Autodesk Inventor part; units mm, degrees
(part 2 of 2)
sketch "スケッチ2" plane through (0, 0, 2.8) normal (0, 0, 1) x (1, 0, 0)
  arc A0 (151.9662, 105.75) -> (150.8837, 107.625) centre (150.8837, 106.375) ccw
  arc A1 (151.9662, 105.75) -> (151.9662, 104.25) centre (153.2652, 105) ccw
  arc A2 (150.8837, 102.375) -> (151.9662, 104.25) centre (150.8837, 103.625) ccw
  arc A3 (147.4196, 101.625) -> (149.5846, 101.625) centre (148.5021, 102.25) ccw
  arc A4 (150.8837, 102.375) -> (149.5846, 101.625) centre (150.8837, 100.875) ccw
  arc A5 (147.4196, 101.625) -> (146.1205, 102.375) centre (146.1205, 100.875) ccw
  arc A6 (146.1205, 107.625) -> (145.038, 105.75) centre (146.1205, 106.375) ccw
  arc A7 (146.1205, 107.625) -> (147.4196, 108.375) centre (146.1205, 109.125) ccw
  line L0 (145.038, 107) -> (148.5021, 109) construction
  circle A8 centre (148.5021, 105) radius 5
  arc A9 (149.5846, 108.375) -> (147.4196, 108.375) centre (148.5021, 107.75) ccw
  arc A10 (145.038, 104.25) -> (145.038, 105.75) centre (143.739, 105) ccw
  arc A11 (149.5846, 108.375) -> (150.8837, 107.625) centre (150.8837, 109.125) ccw
  line L1 (145.038, 103) -> (145.038, 107) construction
  arc A12 (145.038, 104.25) -> (146.1205, 102.375) centre (146.1205, 103.625) ccw
  line L2 (148.5021, 109) -> (151.9662, 107) construction
  line L3 (148.5021, 101) -> (145.038, 103) construction
  circle A13 centre (148.5021, 105) radius 4 construction
  circle A14 centre (148.5021, 105) radius 3.2631 construction
  line L4 (151.9662, 103) -> (148.5021, 101) construction
  line L5 (151.9662, 107) -> (151.9662, 103) construction
  arc A15 (148.8935, 75.5025) -> (149.2852, 76.5042) centre (138.7786, 80.035) ccw projected
  arc A16 (149.2852, 76.5042) -> (149.4997, 77.2537) centre (141.1512, 79.2377) ccw projected
  arc A17 (149.4997, 77.2537) -> (149.5998, 77.772) centre (143.4588, 78.6893) ccw projected
  arc A18 (149.5998, 77.772) -> (150.4063, 77.8165) centre (148.5021, 105) ccw projected
  arc A19 (150.4063, 77.8165) -> (150.5629, 77.3123) centre (156.4092, 79.4038) ccw projected
  arc A20 (150.5629, 77.3123) -> (150.8585, 76.591) centre (158.6424, 80.2027) ccw projected
  arc A21 (150.8585, 76.591) -> (151.358, 75.6385) centre (160.9129, 81.2562) ccw projected
  arc A22 (151.358, 75.6385) -> (152.1361, 75.7246) centre (148.5021, 105) ccw projected
  arc A23 (152.1361, 75.7246) -> (152.4152, 76.7633) centre (141.584, 79.1169) ccw projected
  arc A24 (152.4152, 76.7633) -> (152.546, 77.5318) centre (144.0299, 78.5854) ccw projected
  arc A25 (152.546, 77.5318) -> (152.5884, 78.0581) centre (146.3838, 78.2942) ccw projected
  arc A26 (152.5884, 78.0581) -> (153.3852, 78.191) centre (148.5021, 105) ccw projected
  arc A27 (153.3852, 78.191) -> (153.5962, 77.7071) centre (159.177, 80.429) ccw projected
  arc A28 (153.5962, 77.7071) -> (153.9695, 77.0227) centre (161.3088, 81.4687) ccw projected
  arc A29 (153.9695, 77.0227) -> (154.5707, 76.1309) centre (163.4496, 82.7656) ccw projected
  arc A30 (154.5707, 76.1309) -> (155.3346, 76.3021) centre (148.5021, 105) ccw projected
  arc A31 (155.3346, 76.3021) -> (155.4977, 77.3651) centre (144.4733, 78.5129) ccw projected
  arc A32 (155.4977, 77.3651) -> (155.5431, 78.1434) centre (146.9629, 78.2537) ccw projected
  arc A33 (155.5431, 78.1434) -> (155.5275, 78.6711) centre (149.3345, 78.2232) ccw projected
  arc A34 (155.5275, 78.6711) -> (156.3048, 78.8909) centre (148.5021, 105) ccw projected
  arc A35 (156.3048, 78.8909) -> (156.5678, 78.4331) centre (161.8152, 81.7524) ccw projected
  arc A36 (156.5678, 78.4331) -> (157.014, 77.7939) centre (163.8197, 83.0204) ccw projected
  arc A37 (157.014, 77.7939) -> (157.7097, 76.9737) centre (165.8049, 84.5449) ccw projected
  arc A38 (157.7097, 76.9737) -> (158.4501, 77.2279) centre (148.5021, 105) ccw projected
  arc A39 (158.4501, 77.2279) -> (158.4953, 78.3024) centre (147.4116, 78.2305) ccw projected
  arc A40 (158.4953, 78.3024) -> (158.4549, 79.081) centre (149.9145, 78.2467) ccw projected
  arc A41 (158.4549, 79.081) -> (158.3812, 79.6038) centre (152.2752, 78.4773) ccw projected
  arc A42 (158.3812, 79.6038) -> (159.1296, 79.9077) centre (148.5021, 105) ccw projected
  arc A43 (159.1296, 79.9077) -> (159.4414, 79.4817) centre (164.2918, 83.3581) ccw projected
  arc A44 (159.4414, 79.4817) -> (159.9553, 78.8954) centre (166.1447, 84.8389) ccw projected
  arc A45 (159.9553, 78.8954) -> (160.737, 78.1567) centre (167.9501, 86.5725) ccw projected
  arc A46 (160.737, 78.1567) -> (161.4449, 78.4908) centre (148.5021, 105) ccw projected
  arc A47 (161.4449, 78.4908) -> (161.3716, 79.5638) centre (150.3631, 78.273) ccw projected
  arc A48 (161.3716, 79.5638) -> (161.2458, 80.3332) centre (152.849, 78.5645) ccw projected
  arc A49 (161.2458, 80.3332) -> (161.1151, 80.8447) centre (155.17, 79.0534) ccw projected
  arc A50 (161.1151, 80.8447) -> (161.8255, 81.2291) centre (148.5021, 105) ccw projected
  arc A51 (161.8255, 81.2291) -> (162.1822, 80.84) centre (166.5768, 85.2264) ccw projected
  arc A52 (162.1822, 80.84) -> (162.7575, 80.3138) centre (168.2555, 86.902) ccw projected
  arc A53 (162.7575, 80.3138) -> (163.6157, 79.6656) centre (169.8592, 88.8238) ccw projected
  arc A54 (163.6157, 79.6656) -> (164.2826, 80.0755) centre (148.5021, 105) ccw projected
  arc A55 (164.2826, 80.0755) -> (164.0917, 81.1339) centre (153.292, 78.6399) ccw projected
  arc A56 (164.0917, 81.1339) -> (163.882, 81.8848) centre (155.7308, 79.2031) ccw projected
  arc A57 (163.882, 81.8848) -> (163.6958, 82.3788) centre (157.9838, 79.9444) ccw projected
  arc A58 (163.6958, 82.3788) -> (164.3596, 82.8391) centre (148.5021, 105) ccw projected
  arc A59 (164.3596, 82.8391) -> (164.757, 82.4915) centre (168.6423, 87.3348) ccw projected
  arc A60 (164.757, 82.4915) -> (165.3866, 82.0318) centre (170.1265, 89.1849) ccw projected
  arc A61 (165.3866, 82.0318) -> (166.311, 81.4819) centre (171.5091, 91.2714) ccw projected
  arc A62 (166.311, 81.4819) -> (166.9287, 81.9627) centre (148.5021, 105) ccw projected
  arc A63 (166.9287, 81.9627) -> (166.6226, 82.9938) centre (156.1627, 79.3269) ccw projected
  arc A64 (166.6226, 82.9938) -> (166.3315, 83.717) centre (158.5248, 80.1549) ccw projected
  arc A65 (166.3315, 83.717) -> (166.0921, 84.1875) centre (160.6826, 81.1395) ccw projected
  arc A66 (166.0921, 84.1875) -> (166.7013, 84.7181) centre (148.5021, 105) ccw projected
  arc A67 (166.7013, 84.7181) -> (167.1345, 84.4163) centre (170.4634, 89.6576) ccw projected
  arc A68 (167.1345, 84.4163) -> (167.8108, 84.0287) centre (171.7351, 91.6598) ccw projected
  arc A69 (167.8108, 84.0287) -> (168.7901, 83.5838) centre (172.8797, 93.8857) ccw projected
  arc A70 (168.7901, 83.5838) -> (169.3512, 84.1296) centre (148.5021, 105) ccw projected
  arc A71 (169.3512, 84.1296) -> (168.9334, 85.1207) centre (158.9405, 80.3254) ccw projected
  arc A72 (168.9334, 85.1207) -> (168.5646, 85.8075) centre (161.1971, 81.4083) ccw projected
  arc A73 (168.5646, 85.8075) -> (168.2749, 86.2489) centre (163.2335, 82.6243) ccw projected
  arc A74 (168.2749, 86.2489) -> (168.822, 86.8432) centre (148.5021, 105) ccw projected
  arc A75 (168.822, 86.8432) -> (169.2858, 86.591) centre (172.0179, 92.1667) ccw projected
  arc A76 (169.2858, 86.591) -> (170.0007, 86.2801) centre (173.0616, 94.2966) ccw projected
  arc A77 (170.0007, 86.2801) -> (171.0229, 85.9456) centre (173.9544, 96.6349) ccw projected
  arc A78 (171.0229, 85.9456) -> (171.5205, 86.5499) centre (148.5021, 105) ccw projected
  arc A79 (171.5205, 86.5499) -> (170.9963, 87.489) centre (161.5915, 81.6235) ccw projected
  arc A80 (170.9963, 87.489) -> (170.5541, 88.1311) centre (163.7153, 82.948) ccw projected
  arc A81 (170.5541, 88.1311) -> (170.2177, 88.5379) centre (165.6056, 84.3807) ccw projected
  arc A82 (170.2177, 88.5379) -> (170.6961, 89.1888) centre (148.5021, 105) ccw projected
  arc A83 (170.6961, 89.1888) -> (171.1848, 88.9891) centre (173.287, 94.8315) ccw projected
  arc A84 (171.1848, 88.9891) -> (171.9295, 88.7587) centre (174.09, 97.0633) ccw projected
  arc A85 (171.9295, 88.7587) -> (172.9823, 88.5387) centre (174.7202, 99.4856) ccw projected
  arc A86 (172.9823, 88.5387) -> (173.4105, 89.1941) centre (148.5021, 105) ccw projected
  arc A87 (173.4105, 89.1941) -> (172.7861, 90.0698) centre (164.0837, 83.2053) ccw projected
  arc A88 (172.7861, 90.0698) -> (172.276, 90.6594) centre (166.0489, 84.7555) ccw projected
  arc A89 (172.276, 90.6594) -> (171.8968, 91.0267) centre (167.7701, 86.3874) ccw projected
  arc A90 (171.8968, 91.0267) -> (172.3007, 91.7262) centre (148.5021, 105) ccw projected
  arc A91 (172.3007, 91.7262) -> (172.8084, 91.5815) centre (174.2552, 97.6197) ccw projected
  arc A92 (172.8084, 91.5815) -> (173.574, 91.4345) centre (174.8078, 99.9263) ccw projected
  arc A93 (173.574, 91.4345) -> (174.6446, 91.3317) centre (175.1677, 102.4033) ccw projected
  arc A94 (174.6446, 91.3317) -> (174.9981, 92.0301) centre (148.5021, 105) ccw projected
  arc A95 (174.9981, 92.0301) -> (174.2812, 92.8319) centre (166.3867, 85.0517) ccw projected
  arc A96 (174.2812, 92.8319) -> (173.7093, 93.3617) centre (168.1695, 86.8086) ccw projected
  arc A97 (173.7093, 93.3617) -> (173.292, 93.6851) centre (169.7007, 88.62) ccw projected
  arc A98 (173.292, 93.6851) -> (173.6165, 94.4248) centre (148.5021, 105) ccw projected
  arc A99 (173.6165, 94.4248) -> (174.1371, 94.3369) centre (174.9107, 100.4976) ccw projected
  arc A100 (174.1371, 94.3369) -> (174.9142, 94.275) centre (175.2063, 102.8509) ccw projected
  arc A101 (174.9142, 94.275) -> (175.9896, 94.2905) centre (175.2915, 105.3525) ccw projected
  arc A102 (175.9896, 94.2905) -> (176.2641, 95.0236) centre (148.5021, 105) ccw projected
  arc A103 (176.2641, 95.0236) -> (175.4633, 95.7417) centre (168.4727, 87.1402) ccw projected
  arc A104 (175.4633, 95.7417) -> (174.8366, 96.2054) centre (170.0513, 89.0826) ccw projected
  arc A105 (174.8366, 96.2054) -> (174.3863, 96.4809) centre (171.374, 91.0514) ccw projected
  arc A106 (174.3863, 96.4809) -> (174.6274, 97.2518) centre (148.5021, 105) ccw projected
  arc A107 (174.6274, 97.2518) -> (175.1545, 97.2216) centre (175.2458, 103.4301) ccw projected
  arc A108 (175.1545, 97.2216) -> (175.9337, 97.2456) centre (175.2806, 105.8017) ccw projected
  arc A109 (175.9337, 97.2456) -> (177.0009, 97.3794) centre (175.0901, 108.2974) ccw projected
  arc A110 (177.0009, 97.3794) -> (177.1931, 98.1382) centre (148.5021, 105) ccw projected
  arc A111 (177.1931, 98.1382) -> (176.3182, 98.7638) centre (170.3162, 89.4455) ccw projected
  arc A112 (176.3182, 98.7638) -> (175.6443, 99.1558) centre (171.6716, 91.5498) ccw projected
  arc A113 (175.6443, 99.1558) -> (175.1664, 99.3801) centre (172.7697, 93.6522) ccw projected
  arc A114 (175.1664, 99.3801) -> (175.3212, 100.1729) centre (148.5021, 105) ccw projected
  arc A115 (175.3212, 100.1729) -> (175.8484, 100.2008) centre (175.2562, 106.3816) ccw projected
  arc A116 (175.8484, 100.2008) -> (176.6203, 100.3104) centre (175.0299, 108.7427) ccw projected
  arc A117 (176.6203, 100.3104) -> (177.6663, 100.5607) centre (174.566, 111.2023) ccw projected
  arc A118 (177.6663, 100.5607) -> (177.7738, 101.3361) centre (148.5021, 105) ccw projected
  arc A119 (177.7738, 101.3361) -> (176.8354, 101.8617) centre (171.8949, 91.9397) ccw projected
  arc A120 (176.8354, 101.8617) -> (176.1225, 102.1771) centre (173.0106, 94.1803) ccw projected
  arc A121 (176.1225, 102.1771) -> (175.6228, 102.3475) centre (173.8707, 96.3907) ccw projected
  arc A122 (175.6228, 102.3475) -> (175.6895, 103.1525) centre (148.5021, 105) ccw projected
  arc A123 (175.6895, 103.1525) -> (176.2104, 103.2383) centre (174.9418, 109.3164) ccw projected
  arc A124 (176.2104, 103.2383) -> (176.9655, 103.4321) centre (174.4572, 111.6382) ccw projected
  arc A125 (176.9655, 103.4321) -> (177.9776, 103.796) centre (173.7255, 114.0319) ccw projected
  arc A126 (177.9776, 103.796) -> (177.9992, 104.5785) centre (148.5021, 105) ccw projected
  arc A127 (177.9992, 104.5785) -> (177.0087, 104.9976) centre (173.1897, 94.5923) ccw projected
  arc A128 (177.0087, 104.9976) -> (176.2654, 105.2327) centre (174.0521, 96.9421) ccw projected
  arc A129 (176.2654, 105.2327) -> (175.75, 105.3471) centre (174.6639, 99.2337) ccw projected
  arc A130 (175.75, 105.3471) -> (175.7277, 106.1545) centre (148.5021, 105) ccw projected
  arc A131 (175.7277, 106.1545) -> (176.236, 106.2971) centre (174.3065, 112.1988) ccw projected
  arc A132 (176.236, 106.2971) -> (176.9653, 106.5728) centre (173.5694, 114.4532) ccw projected
  arc A133 (176.9653, 106.5728) -> (177.9312, 107.0458) centre (172.5788, 116.7519) ccw projected
  arc A134 (177.9312, 107.0458) -> (177.8665, 107.826) centre (148.5021, 105) ccw projected
  arc A135 (177.8665, 107.826) -> (176.8359, 108.1336) centre (174.1848, 97.3713) ccw projected
  arc A136 (176.8359, 108.1336) -> (176.0713, 108.2855) centre (174.7835, 99.8017) ccw projected
  arc A137 (176.0713, 108.2855) -> (175.5464, 108.3424) centre (175.1394, 102.1467) ccw projected
  arc A138 (175.5464, 108.3424) -> (175.4355, 109.1426) centre (148.5021, 105) ccw projected
  arc A139 (175.4355, 109.1426) -> (175.925, 109.3402) centre (173.3579, 114.9938) ccw projected
  arc A140 (175.925, 109.3402) -> (176.6195, 109.6944) centre (172.3773, 117.1534) ccw projected
  arc A141 (176.6195, 109.6944) -> (177.5275, 110.2709) centre (171.1399, 119.3292) ccw projected
  arc A142 (177.5275, 110.2709) -> (177.3774, 111.0391) centre (148.5021, 105) ccw projected
  arc A143 (177.3774, 111.0391) -> (176.3192, 111.2315) centre (174.8681, 100.2429) ccw projected
  arc A144 (176.3192, 111.2315) -> (175.5425, 111.2984) centre (175.1958, 102.7244) ccw projected
  arc A145 (175.5425, 111.2984) -> (175.0146, 111.2973) centre (175.2916, 105.0943) ccw projected
  arc A146 (175.0146, 111.2973) -> (174.8163, 112.0803) centre (148.5021, 105) ccw projected
  arc A147 (174.8163, 112.0803) -> (175.2811, 112.3306) centre (172.1077, 117.6675) ccw projected
  arc A148 (175.2811, 112.3306) -> (175.9324, 112.7591) centre (170.8954, 119.7062) ccw projected
  arc A149 (175.9324, 112.7591) -> (176.7715, 113.4319) centre (169.4262, 121.7326) ccw projected
  arc A150 (176.7715, 113.4319) -> (176.5378, 114.179) centre (148.5021, 105) ccw projected
  arc A151 (176.5378, 114.179) -> (175.4649, 114.2538) centre (175.2314, 103.1723) ccw projected
  arc A152 (175.4649, 114.2538) -> (174.6855, 114.2348) centre (175.2841, 105.6748) ccw projected
  arc A153 (174.6855, 114.2348) -> (174.1609, 114.1756) centre (175.1187, 108.0408) ccw projected
  arc A154 (174.1609, 114.1756) -> (173.8777, 114.9321) centre (148.5021, 105) ccw projected
  arc A155 (173.8777, 114.9321) -> (174.3122, 115.232) centre (170.5709, 120.1874) ccw projected
  arc A156 (174.3122, 115.232) -> (174.9124, 115.7295) centre (169.1417, 122.0803) ccw projected
  arc A157 (174.9124, 115.7295) -> (175.6723, 116.4906) centre (167.4585, 123.9328) ccw projected
  arc A158 (175.6723, 116.4906) -> (175.3579, 117.2075) centre (148.5021, 105) ccw projected
  arc A159 (175.3579, 117.2075) -> (174.2833, 117.1638) centre (175.2702, 106.1238) ccw projected
  arc A160 (174.2833, 117.1638) -> (173.5107, 117.0592) centre (175.0474, 108.6169) ccw projected
  arc A161 (173.5107, 117.0592) -> (172.9958, 116.9426) centre (174.6226, 110.9504) ccw projected
  arc A162 (172.9958, 116.9426) -> (172.6311, 117.6634) centre (148.5021, 105) ccw projected
  arc A163 (172.6311, 117.6634) -> (173.0299, 118.0092) centre (168.7662, 122.523) ccw projected
  arc A164 (173.0299, 118.0092) -> (173.5717, 118.5698) centre (167.1375, 124.2472) ccw projected
  arc A165 (173.5717, 118.5698) -> (174.2434, 119.4098) centre (165.2607, 125.9033) ccw projected
  arc A166 (174.2434, 119.4098) -> (173.852, 120.0877) centre (148.5021, 105) ccw projected
  arc A167 (173.852, 120.0877) -> (172.7887, 119.9261) centre (174.9841, 109.0617) ccw projected
  arc A168 (172.7887, 119.9261) -> (172.0323, 119.7371) centre (174.4884, 111.5151) ccw projected
  arc A169 (172.0323, 119.7371) -> (171.5334, 119.5646) centre (173.8095, 113.7878) ccw projected
  arc A170 (171.5334, 119.5646) -> (171.0916, 120.2409) centre (148.5021, 105) ccw projected
  arc A171 (171.0916, 120.2409) -> (171.4499, 120.6285) centre (166.7155, 124.6458) ccw projected
  arc A172 (171.4499, 120.6285) -> (171.9268, 121.2453) centre (164.907, 126.1804) ccw projected
  arc A173 (171.9268, 121.2453) -> (172.502, 122.1541) centre (162.8594, 127.62) ccw projected
  arc A174 (172.502, 122.1541) -> (172.0384, 122.7849) centre (148.5021, 105) ccw projected
  arc A175 (172.0384, 122.7849) -> (170.9993, 122.5072) centre (174.3766, 111.9503) ccw projected
  arc A176 (170.9993, 122.5072) -> (170.2683, 122.2362) centre (173.6139, 114.3343) ccw projected
  arc A177 (170.2683, 122.2362) -> (169.7913, 122.0099) centre (172.6892, 116.5185) ccw projected
  arc A178 (169.7913, 122.0099) -> (169.2778, 122.6334) centre (148.5021, 105) ccw projected
  arc A179 (169.2778, 122.6334) -> (169.5914, 123.0581) centre (164.4438, 126.5302) ccw projected
  arc A180 (169.5914, 123.0581) -> (169.9975, 123.7236) centre (162.4774, 127.8566) ccw projected
  arc A181 (169.9975, 123.7236) -> (170.4692, 124.6902) centre (160.2839, 129.0621) ccw projected
  arc A182 (170.4692, 124.6902) -> (169.939, 125.2661) centre (148.5021, 105) ccw projected
  arc A183 (169.939, 125.2661) -> (168.9368, 124.8758) centre (173.455, 114.7545) ccw projected
  arc A184 (168.9368, 124.8758) -> (168.2401, 124.526) centre (172.4347, 117.0402) ccw projected
  arc A185 (168.2401, 124.526) -> (167.7909, 124.2486) centre (171.2752, 119.1093) ccw projected
  arc A186 (167.7909, 124.2486) -> (167.2119, 124.8119) centre (148.5021, 105) ccw projected
  arc A187 (167.2119, 124.8119) -> (167.4768, 125.2685) centre (161.9785, 128.1533) ccw projected
  arc A188 (167.4768, 125.2685) -> (167.8073, 125.9746) centre (159.8782, 129.2552) ccw projected
  arc A189 (167.8073, 125.9746) -> (168.1698, 126.9872) centre (157.5654, 130.2122) ccw projected
  arc A190 (168.1698, 126.9872) -> (167.5795, 127.5013) centre (148.5021, 105) ccw projected
  arc A191 (167.5795, 127.5013) -> (166.6263, 127.0032) centre (172.2304, 117.4404) ccw projected
  arc A192 (166.6263, 127.0032) -> (165.9723, 126.5789) centre (170.9649, 119.5999) ccw projected
  arc A193 (165.9723, 126.5789) -> (165.5563, 126.2537) centre (169.5849, 121.5289) ccw projected
  arc A194 (165.5563, 126.2537) -> (164.9189, 126.7499) centre (148.5021, 105) ccw projected
  arc A195 (164.9189, 126.7499) -> (165.132, 127.2329) centre (159.3497, 129.4953) ccw projected
  arc A196 (165.132, 127.2329) -> (165.3828, 127.971) centre (157.1409, 130.3595) ccw projected
  arc A197 (165.3828, 127.971) -> (165.6317, 129.0174) centre (154.7368, 131.0562) ccw projected
  arc A198 (165.6317, 129.0174) -> (164.9884, 129.4634) centre (148.5021, 105) ccw projected
  arc A199 (164.9884, 129.4634) -> (164.0957, 128.8635) centre (170.7179, 119.9752) ccw projected
  arc A200 (164.0957, 128.8635) -> (163.4924, 128.3698) centre (169.2225, 121.9823) ccw projected
  arc A201 (163.4924, 128.3698) -> (163.1147, 128.0008) centre (167.6386, 123.7479) ccw projected
  arc A202 (163.1147, 128.0008) -> (162.4266, 128.4239) centre (148.5021, 105) ccw projected
  arc A203 (162.4266, 128.4239) -> (162.5852, 128.9274) centre (156.5892, 130.5399) ccw projected
  arc A204 (162.5852, 128.9274) -> (162.7533, 129.6886) centre (154.2987, 131.1559) ccw projected
  arc A205 (162.7533, 129.6886) -> (162.8856, 130.756) centre (151.8326, 131.5839) ccw projected
  arc A206 (162.8856, 130.756) -> (162.1971, 131.1286) centre (148.5021, 105) ccw projected
  arc A207 (162.1971, 131.1286) -> (161.3759, 130.434) centre (168.9357, 122.3282) ccw projected
  arc A208 (161.3759, 130.434) -> (160.8305, 129.877) centre (167.2285, 124.1587) ccw projected
  arc A209 (160.8305, 129.877) -> (160.4958, 129.4688) centre (165.46, 125.7393) ccw projected
  arc A210 (160.4958, 129.4688) -> (159.7653, 129.8135) centre (148.5021, 105) ccw projected
  arc A211 (159.7653, 129.8135) -> (159.8676, 130.3314) centre (153.7305, 131.2746) ccw projected
  arc A212 (159.8676, 130.3314) -> (159.9509, 131.1065) centre (151.3862, 131.6349) ccw projected
  arc A213 (159.9509, 131.1065) -> (159.9649, 132.182) centre (148.8879, 131.789) ccw projected
  arc A214 (159.9649, 132.182) -> (159.2397, 132.4766) centre (148.5021, 105) ccw projected
  arc A215 (159.2397, 132.4766) -> (158.4998, 131.6959) centre (166.9054, 124.4709) ccw projected
  arc A216 (158.4998, 131.6959) -> (158.019, 131.0822) centre (165.0072, 126.1025) ccw projected
  arc A217 (158.019, 131.0822) -> (157.7312, 130.6397) centre (163.0756, 127.4789) ccw projected
  arc A218 (157.7312, 130.6397) -> (156.9672, 130.9019) centre (148.5021, 105) ccw projected
  arc A219 (156.9672, 130.9019) -> (157.0119, 131.428) centre (150.8084, 131.6903) ccw projected
  arc A220 (157.0119, 131.428) -> (157.0094, 132.2076) centre (148.4386, 131.7905) ccw projected
  arc A221 (157.0094, 132.2076) -> (156.9051, 133.278) centre (145.9386, 131.6688) ccw projected
  arc A222 (156.9051, 133.278) -> (156.1518, 133.491) centre (148.5021, 105) ccw projected
  arc A223 (156.1518, 133.491) -> (155.5024, 132.6337) centre (164.6518, 126.3772) ccw projected
  arc A224 (155.5024, 132.6337) -> (155.092, 131.9709) centre (162.5856, 127.7901) ccw projected
  arc A225 (155.092, 131.9709) -> (154.8546, 131.4993) centre (160.5143, 128.9457) ccw projected
  arc A226 (154.8546, 131.4993) -> (154.0664, 131.676) centre (148.5021, 105) ccw projected
  arc A227 (154.0664, 131.676) -> (154.053, 132.2037) centre (147.8582, 131.782) ccw projected
  arc A228 (154.053, 132.2037) -> (153.9648, 132.9783) centre (145.4918, 131.6209) ccw projected
  arc A229 (153.9648, 132.9783) -> (153.7433, 134.0308) centre (143.0203, 131.2249) ccw projected
  arc A230 (153.7433, 134.0308) -> (152.9711, 134.1596) centre (148.5021, 105) ccw projected
  arc A231 (152.9711, 134.1596) -> (152.4201, 133.2365) centre (162.202, 128.0241) ccw projected
  arc A232 (152.4201, 133.2365) -> (152.0848, 132.5318) centre (159.993, 129.2012) ccw projected
  arc A233 (152.0848, 132.5318) -> (151.9009, 132.0373) centre (157.8071, 130.1218) ccw projected
  arc A234 (151.9009, 132.0373) -> (151.098, 132.1262) centre (148.5021, 105) ccw projected
  arc A235 (151.098, 132.1262) -> (151.0266, 132.6493) centre (144.9158, 131.5487) ccw projected
  arc A236 (151.0266, 132.6493) -> (150.8537, 133.4095) centre (142.5815, 131.1282) ccw projected
  arc A237 (150.8537, 133.4095) -> (150.5178, 134.4312) centre (140.1686, 130.4628) ccw projected
  arc A238 (150.5178, 134.4312) -> (149.7362, 134.4743) centre (148.5021, 105) ccw projected
  arc A239 (149.7362, 134.4743) -> (149.29, 133.4958) centre (159.5861, 129.3914) ccw projected
  arc A240 (149.29, 133.4958) -> (149.0345, 132.7592) centre (157.261, 130.3183) ccw projected
  arc A241 (149.0345, 132.7592) -> (148.906, 132.2471) centre (154.9871, 130.993) ccw projected
  arc A242 (148.906, 132.2471) -> (148.0982, 132.2471) centre (148.5021, 105) ccw projected
  arc A243 (148.0982, 132.2471) -> (147.9697, 132.7592) centre (142.0171, 130.9929) ccw projected
  arc A244 (147.9697, 132.7592) -> (147.7142, 133.4957) centre (139.7432, 130.3183) ccw projected
  arc A245 (147.7142, 133.4957) -> (147.2679, 134.4743) centre (137.4181, 129.3914) ccw projected
  arc A246 (147.2679, 134.4743) -> (146.4863, 134.4312) centre (148.5021, 105) ccw projected
  arc A247 (146.4863, 134.4312) -> (146.1504, 133.4094) centre (156.8355, 130.4627) ccw projected
  arc A248 (146.1504, 133.4094) -> (145.9775, 132.6493) centre (154.4226, 131.1282) ccw projected
  arc A249 (145.9775, 132.6493) -> (145.9061, 132.1262) centre (152.0883, 131.5486) ccw projected
  arc A250 (145.9061, 132.1262) -> (145.1033, 132.0373) centre (148.5021, 105) ccw projected
  arc A251 (145.1033, 132.0373) -> (144.9192, 132.5321) centre (139.197, 130.1218) ccw projected
  arc A252 (144.9192, 132.5321) -> (144.5842, 133.2361) centre (137.0111, 129.2011) ccw projected
  arc A253 (144.5842, 133.2361) -> (144.033, 134.1596) centre (134.8021, 128.0241) ccw projected
  arc A254 (144.033, 134.1596) -> (143.2609, 134.0308) centre (148.5021, 105) ccw projected
  arc A255 (143.2609, 134.0308) -> (143.0394, 132.9783) centre (153.9839, 131.2249) ccw projected
  arc A256 (143.0394, 132.9783) -> (142.9512, 132.2037) centre (151.5124, 131.6209) ccw projected
  arc A257 (142.9512, 132.2037) -> (142.9378, 131.676) centre (149.146, 131.782) ccw projected
  arc A258 (142.9378, 131.676) -> (142.1496, 131.4993) centre (148.5021, 105) ccw projected
  arc A259 (142.1496, 131.4993) -> (141.9122, 131.9709) centre (136.4899, 128.9457) ccw projected
  arc A260 (141.9122, 131.9709) -> (141.5018, 132.6337) centre (134.4186, 127.7901) ccw projected
  arc A261 (141.5018, 132.6337) -> (140.8524, 133.491) centre (132.3524, 126.3772) ccw projected
  arc A262 (140.8524, 133.491) -> (140.0991, 133.278) centre (148.5021, 105) ccw projected
  arc A263 (140.0991, 133.278) -> (139.9947, 132.2076) centre (151.0656, 131.6688) ccw projected
  arc A264 (139.9947, 132.2076) -> (139.9923, 131.428) centre (148.5656, 131.7905) ccw projected
  arc A265 (139.9923, 131.428) -> (140.037, 130.9019) centre (146.1958, 131.6903) ccw projected
  arc A266 (140.037, 130.9019) -> (139.273, 130.6397) centre (148.5021, 105) ccw projected
  arc A267 (139.273, 130.6397) -> (138.9852, 131.0822) centre (133.9286, 127.4789) ccw projected
  arc A268 (138.9852, 131.0822) -> (138.5044, 131.6959) centre (131.997, 126.1025) ccw projected
  arc A269 (138.5044, 131.6959) -> (137.7645, 132.4766) centre (130.0988, 124.4709) ccw projected
  arc A270 (137.7645, 132.4766) -> (137.0393, 132.182) centre (148.5021, 105) ccw projected
  arc A271 (137.0393, 132.182) -> (137.0533, 131.1065) centre (148.1163, 131.789) ccw projected
  arc A272 (137.0533, 131.1065) -> (137.1366, 130.3314) centre (145.618, 131.6349) ccw projected
  arc A273 (137.1366, 130.3314) -> (137.2389, 129.8135) centre (143.2737, 131.2746) ccw projected
  arc A274 (137.2389, 129.8135) -> (136.5084, 129.4688) centre (148.5021, 105) ccw projected
  arc A275 (136.5084, 129.4688) -> (136.1737, 129.877) centre (131.5441, 125.7393) ccw projected
  arc A276 (136.1737, 129.877) -> (135.6283, 130.434) centre (129.7757, 124.1587) ccw projected
  arc A277 (135.6283, 130.434) -> (134.8071, 131.1286) centre (128.0685, 122.3282) ccw projected
  arc A278 (134.8071, 131.1286) -> (134.1186, 130.756) centre (148.5021, 105) ccw projected
  arc A279 (134.1186, 130.756) -> (134.2509, 129.6886) centre (145.1716, 131.5839) ccw projected
  arc A280 (134.2509, 129.6886) -> (134.4189, 128.9274) centre (142.7055, 131.1559) ccw projected
  arc A281 (134.4189, 128.9274) -> (134.5776, 128.4239) centre (140.415, 130.5399) ccw projected
  arc A282 (134.5776, 128.4239) -> (133.8894, 128.0008) centre (148.5021, 105) ccw projected
  arc A283 (133.8894, 128.0008) -> (133.5118, 128.3698) centre (129.3656, 123.7479) ccw projected
  arc A284 (133.5118, 128.3698) -> (132.9085, 128.8635) centre (127.7817, 121.9823) ccw projected
  arc A285 (132.9085, 128.8635) -> (132.0158, 129.4634) centre (126.2863, 119.9752) ccw projected
  arc A286 (132.0158, 129.4634) -> (131.3725, 129.0174) centre (148.5021, 105) ccw projected
  arc A287 (131.3725, 129.0174) -> (131.6214, 127.971) centre (142.2674, 131.0562) ccw projected
  arc A288 (131.6214, 127.971) -> (131.8722, 127.2329) centre (139.8633, 130.3595) ccw projected
  arc A289 (131.8722, 127.2329) -> (132.0853, 126.7499) centre (137.6545, 129.4953) ccw projected
  arc A290 (132.0853, 126.7499) -> (131.4479, 126.2537) centre (148.5021, 105) ccw projected
  arc A291 (131.4479, 126.2537) -> (131.0319, 126.5789) centre (127.4193, 121.5289) ccw projected
  arc A292 (131.0319, 126.5789) -> (130.3779, 127.0032) centre (126.0393, 119.5999) ccw projected
  arc A293 (130.3779, 127.0032) -> (129.4247, 127.5013) centre (124.7737, 117.4403) ccw projected
  arc A294 (129.4247, 127.5013) -> (128.8344, 126.9872) centre (148.5021, 105) ccw projected
  arc A295 (128.8344, 126.9872) -> (129.1969, 125.9746) centre (139.4388, 130.2122) ccw projected
  arc A296 (129.1969, 125.9746) -> (129.5273, 125.2685) centre (137.126, 129.2552) ccw projected
  arc A297 (129.5273, 125.2685) -> (129.7923, 124.8119) centre (135.0256, 128.1533) ccw projected
  arc A298 (129.7923, 124.8119) -> (129.2133, 124.2486) centre (148.5021, 105) ccw projected
  arc A299 (129.2133, 124.2486) -> (128.7641, 124.526) centre (125.7289, 119.1093) ccw projected
  arc A300 (128.7641, 124.526) -> (128.0674, 124.8758) centre (124.5695, 117.0402) ccw projected
  arc A301 (128.0674, 124.8758) -> (127.0652, 125.2661) centre (123.5492, 114.7545) ccw projected
  arc A302 (127.0652, 125.2661) -> (126.535, 124.6902) centre (148.5021, 105) ccw projected
  arc A303 (126.535, 124.6902) -> (127.0067, 123.7236) centre (136.7203, 129.0621) ccw projected
  arc A304 (127.0067, 123.7236) -> (127.4128, 123.0581) centre (134.5267, 127.8566) ccw projected
  arc A305 (127.4128, 123.0581) -> (127.7264, 122.6334) centre (132.5604, 126.5302) ccw projected
  arc A306 (127.7264, 122.6334) -> (127.2128, 122.0099) centre (148.5021, 105) ccw projected
  arc A307 (127.2128, 122.0099) -> (126.7359, 122.2362) centre (124.315, 116.5185) ccw projected
  arc A308 (126.7359, 122.2362) -> (126.0049, 122.5072) centre (123.3903, 114.3343) ccw projected
  arc A309 (126.0049, 122.5072) -> (124.9658, 122.7849) centre (122.6276, 111.9503) ccw projected
  arc A310 (124.9658, 122.7849) -> (124.5022, 122.1541) centre (148.5021, 105) ccw projected
  arc A311 (124.5022, 122.1541) -> (125.0774, 121.2453) centre (134.1448, 127.62) ccw projected
  arc A312 (125.0774, 121.2453) -> (125.5543, 120.6285) centre (132.0972, 126.1804) ccw projected
  arc A313 (125.5543, 120.6285) -> (125.9126, 120.2409) centre (130.2886, 124.6458) ccw projected
  arc A314 (125.9126, 120.2409) -> (125.4708, 119.5646) centre (148.5021, 105) ccw projected
  arc A315 (125.4708, 119.5646) -> (124.9719, 119.7371) centre (123.1947, 113.7878) ccw projected
  arc A316 (124.9719, 119.7371) -> (124.2155, 119.9261) centre (122.5158, 111.5151) ccw projected
  arc A317 (124.2155, 119.9261) -> (123.1522, 120.0877) centre (122.02, 109.0617) ccw projected
  arc A318 (123.1522, 120.0877) -> (122.7608, 119.4098) centre (148.5021, 105) ccw projected
  arc A319 (122.7608, 119.4098) -> (123.4325, 118.5698) centre (131.7435, 125.9033) ccw projected
  arc A320 (123.4325, 118.5698) -> (123.9743, 118.0092) centre (129.8667, 124.2472) ccw projected
  arc A321 (123.9743, 118.0092) -> (124.3731, 117.6634) centre (128.238, 122.523) ccw projected
  arc A322 (124.3731, 117.6634) -> (124.0084, 116.9426) centre (148.5021, 105) ccw projected
  arc A323 (124.0084, 116.9426) -> (123.4935, 117.0592) centre (122.3816, 110.9504) ccw projected
  arc A324 (123.4935, 117.0592) -> (122.7209, 117.1638) centre (121.9568, 108.6169) ccw projected
  arc A325 (122.7209, 117.1638) -> (121.6463, 117.2075) centre (121.734, 106.1238) ccw projected
  arc A326 (121.6463, 117.2075) -> (121.3318, 116.4906) centre (148.5021, 105) ccw projected
  arc A327 (121.3318, 116.4906) -> (122.0918, 115.7295) centre (129.5457, 123.9328) ccw projected
  arc A328 (122.0918, 115.7295) -> (122.692, 115.232) centre (127.8625, 122.0803) ccw projected
  arc A329 (122.692, 115.232) -> (123.1265, 114.9321) centre (126.4333, 120.1874) ccw projected
  arc A330 (123.1265, 114.9321) -> (122.8433, 114.1756) centre (148.5021, 105) ccw projected
  arc A331 (122.8433, 114.1756) -> (122.3187, 114.2348) centre (121.8855, 108.0408) ccw projected
  arc A332 (122.3187, 114.2348) -> (121.5393, 114.2538) centre (121.7201, 105.6747) ccw projected
  arc A333 (121.5393, 114.2538) -> (120.4664, 114.179) centre (121.7728, 103.1723) ccw projected
  arc A334 (120.4664, 114.179) -> (120.2327, 113.4319) centre (148.5021, 105) ccw projected
  arc A335 (120.2327, 113.4319) -> (121.0718, 112.7591) centre (127.578, 121.7326) ccw projected
  arc A336 (121.0718, 112.7591) -> (121.7231, 112.3306) centre (126.1087, 119.7061) ccw projected
  arc A337 (121.7231, 112.3306) -> (122.1879, 112.0803) centre (124.8965, 117.6675) ccw projected
  arc A338 (122.1879, 112.0803) -> (121.9896, 111.2973) centre (148.5021, 105) ccw projected
  arc A339 (121.9896, 111.2973) -> (121.4617, 111.2984) centre (121.7126, 105.0943) ccw projected
  arc A340 (121.4617, 111.2984) -> (120.685, 111.2315) centre (121.8084, 102.7244) ccw projected
  arc A341 (120.685, 111.2315) -> (119.6268, 111.0391) centre (122.1361, 100.2429) ccw projected
  arc A342 (119.6268, 111.0391) -> (119.4767, 110.2709) centre (148.5021, 105) ccw projected
  arc A343 (119.4767, 110.2709) -> (120.3847, 109.6944) centre (125.8643, 119.3292) ccw projected
  arc A344 (120.3847, 109.6944) -> (121.0792, 109.3402) centre (124.6269, 117.1534) ccw projected
  arc A345 (121.0792, 109.3402) -> (121.5687, 109.1426) centre (123.6463, 114.9938) ccw projected
  arc A346 (121.5687, 109.1426) -> (121.4578, 108.3424) centre (148.5021, 105) ccw projected
  arc A347 (121.4578, 108.3424) -> (120.9329, 108.2855) centre (121.8648, 102.1467) ccw projected
  arc A348 (120.9329, 108.2855) -> (120.1683, 108.1336) centre (122.2207, 99.8017) ccw projected
  arc A349 (120.1683, 108.1336) -> (119.1377, 107.826) centre (122.8194, 97.3713) ccw projected
  arc A350 (119.1377, 107.826) -> (119.073, 107.0458) centre (148.5021, 105) ccw projected
  arc A351 (119.073, 107.0458) -> (120.0389, 106.5728) centre (124.4253, 116.7519) ccw projected
  arc A352 (120.0389, 106.5728) -> (120.7682, 106.2971) centre (123.4348, 114.4532) ccw projected
  arc A353 (120.7682, 106.2971) -> (121.2765, 106.1545) centre (122.6977, 112.1988) ccw projected
  arc A354 (121.2765, 106.1545) -> (121.2542, 105.3471) centre (148.5021, 105) ccw projected
  arc A355 (121.2542, 105.3471) -> (120.7388, 105.2327) centre (122.3403, 99.2337) ccw projected
  arc A356 (120.7388, 105.2327) -> (119.9955, 104.9976) centre (122.9521, 96.9421) ccw projected
  arc A357 (119.9955, 104.9976) -> (119.005, 104.5785) centre (123.8145, 94.5923) ccw projected
  arc A358 (119.005, 104.5785) -> (119.0266, 103.796) centre (148.5021, 105) ccw projected
  arc A359 (119.0266, 103.796) -> (120.0387, 103.4321) centre (123.2787, 114.0319) ccw projected
  arc A360 (120.0387, 103.4321) -> (120.7938, 103.2383) centre (122.547, 111.6382) ccw projected
  arc A361 (120.7938, 103.2383) -> (121.3147, 103.1525) centre (122.0624, 109.3164) ccw projected
  arc A362 (121.3147, 103.1525) -> (121.3814, 102.3475) centre (148.5021, 105) ccw projected
  arc A363 (121.3814, 102.3475) -> (120.8817, 102.1771) centre (123.1335, 96.3907) ccw projected
  arc A364 (120.8817, 102.1771) -> (120.1688, 101.8617) centre (123.9936, 94.1803) ccw projected
  arc A365 (120.1688, 101.8617) -> (119.2304, 101.3361) centre (125.1093, 91.9397) ccw projected
  arc A366 (119.2304, 101.3361) -> (119.3379, 100.5607) centre (148.5021, 105) ccw projected
  arc A367 (119.3379, 100.5607) -> (120.3839, 100.3104) centre (122.4382, 111.2023) ccw projected
  arc A368 (120.3839, 100.3104) -> (121.1558, 100.2008) centre (121.9743, 108.7427) ccw projected
  arc A369 (121.1558, 100.2008) -> (121.683, 100.1728) centre (121.748, 106.3816) ccw projected
  arc A370 (121.683, 100.1728) -> (121.8378, 99.3801) centre (148.5021, 105) ccw projected
  arc A371 (121.8378, 99.3801) -> (121.3599, 99.1558) centre (124.2345, 93.6522) ccw projected
  arc A372 (121.3599, 99.1558) -> (120.686, 98.7638) centre (125.3326, 91.5498) ccw projected
  arc A373 (120.686, 98.7638) -> (119.8111, 98.1382) centre (126.688, 89.4455) ccw projected
  arc A374 (119.8111, 98.1382) -> (120.0033, 97.3794) centre (148.5021, 105) ccw projected
  arc A375 (120.0033, 97.3794) -> (121.0705, 97.2456) centre (121.9141, 108.2974) ccw projected
  arc A376 (121.0705, 97.2456) -> (121.8497, 97.2216) centre (121.7236, 105.8017) ccw projected
  arc A377 (121.8497, 97.2216) -> (122.3768, 97.2518) centre (121.7584, 103.4301) ccw projected
  arc A378 (122.3768, 97.2518) -> (122.6179, 96.4809) centre (148.5021, 105) ccw projected
  arc A379 (122.6179, 96.4809) -> (122.1676, 96.2054) centre (125.6302, 91.0514) ccw projected
  arc A380 (122.1676, 96.2054) -> (121.5409, 95.7417) centre (126.9529, 89.0826) ccw projected
  arc A381 (121.5409, 95.7417) -> (120.7401, 95.0236) centre (128.5315, 87.1402) ccw projected
  arc A382 (120.7401, 95.0236) -> (121.0146, 94.2905) centre (148.5021, 105) ccw projected
  arc A383 (121.0146, 94.2905) -> (122.09, 94.2749) centre (121.7127, 105.3525) ccw projected
  arc A384 (122.09, 94.2749) -> (122.8671, 94.3369) centre (121.7979, 102.8509) ccw projected
  arc A385 (122.8671, 94.3369) -> (123.3877, 94.4248) centre (122.0935, 100.4976) ccw projected
  arc A386 (123.3877, 94.4248) -> (123.7122, 93.6851) centre (148.5021, 105) ccw projected
  arc A387 (123.7122, 93.6851) -> (123.2949, 93.3617) centre (127.3035, 88.62) ccw projected
  arc A388 (123.2949, 93.3617) -> (122.723, 92.8319) centre (128.8347, 86.8086) ccw projected
  arc A389 (122.723, 92.8319) -> (122.0061, 92.0301) centre (130.6175, 85.0517) ccw projected
  arc A390 (122.0061, 92.0301) -> (122.3596, 91.3317) centre (148.5021, 105) ccw projected
  arc A391 (122.3596, 91.3317) -> (123.4302, 91.4345) centre (121.8365, 102.4033) ccw projected
  arc A392 (123.4302, 91.4345) -> (124.1958, 91.5815) centre (122.1964, 99.9263) ccw projected
  arc A393 (124.1958, 91.5815) -> (124.7035, 91.7262) centre (122.749, 97.6197) ccw projected
  arc A394 (124.7035, 91.7262) -> (125.1074, 91.0267) centre (148.5021, 105) ccw projected
  arc A395 (125.1074, 91.0267) -> (124.7282, 90.6594) centre (129.2341, 86.3874) ccw projected
  arc A396 (124.7282, 90.6594) -> (124.218, 90.0698) centre (130.9553, 84.7555) ccw projected
  arc A397 (124.218, 90.0698) -> (123.5937, 89.1941) centre (132.9205, 83.2053) ccw projected
  arc A398 (123.5937, 89.1941) -> (124.0219, 88.5387) centre (148.5021, 105) ccw projected
  arc A399 (124.0219, 88.5387) -> (125.0747, 88.7587) centre (122.284, 99.4856) ccw projected
  arc A400 (125.0747, 88.7587) -> (125.8194, 88.9891) centre (122.9142, 97.0633) ccw projected
  arc A401 (125.8194, 88.9891) -> (126.3081, 89.1888) centre (123.7172, 94.8315) ccw projected
  arc A402 (126.3081, 89.1888) -> (126.7865, 88.5379) centre (148.5021, 105) ccw projected
  arc A403 (126.7865, 88.5379) -> (126.4501, 88.1311) centre (131.3985, 84.3807) ccw projected
  arc A404 (126.4501, 88.1311) -> (126.0079, 87.489) centre (133.2889, 82.948) ccw projected
  arc A405 (126.0079, 87.489) -> (125.4837, 86.5499) centre (135.4127, 81.6235) ccw projected
  arc A406 (125.4837, 86.5499) -> (125.9813, 85.9456) centre (148.5021, 105) ccw projected
  arc A407 (125.9813, 85.9456) -> (127.0035, 86.2801) centre (123.0498, 96.6349) ccw projected
  arc A408 (127.0035, 86.2801) -> (127.7184, 86.591) centre (123.9426, 94.2965) ccw projected
  arc A409 (127.7184, 86.591) -> (128.1822, 86.8432) centre (124.9863, 92.1667) ccw projected
  arc A410 (128.1822, 86.8432) -> (128.7293, 86.2489) centre (148.5021, 105) ccw projected
  arc A411 (128.7293, 86.2489) -> (128.4396, 85.8076) centre (133.7707, 82.6243) ccw projected
  arc A412 (128.4396, 85.8076) -> (128.0708, 85.1207) centre (135.8071, 81.4083) ccw projected
  arc A413 (128.0708, 85.1207) -> (127.653, 84.1296) centre (138.0637, 80.3254) ccw projected
  arc A414 (127.653, 84.1296) -> (128.2141, 83.5838) centre (148.5021, 105) ccw projected
  arc A415 (128.2141, 83.5838) -> (129.1933, 84.0287) centre (124.1245, 93.8857) ccw projected
  arc A416 (129.1933, 84.0287) -> (129.8697, 84.4163) centre (125.2691, 91.6598) ccw projected
  arc A417 (129.8697, 84.4163) -> (130.3029, 84.7181) centre (126.5408, 89.6576) ccw projected
  arc A418 (130.3029, 84.7181) -> (130.9121, 84.1875) centre (148.5021, 105) ccw projected
  arc A419 (130.9121, 84.1875) -> (130.6727, 83.717) centre (136.3216, 81.1395) ccw projected
  arc A420 (130.6727, 83.717) -> (130.3816, 82.9938) centre (138.4794, 80.1549) ccw projected
  arc A421 (130.3816, 82.9938) -> (130.0755, 81.9627) centre (140.8415, 79.3269) ccw projected
  arc A422 (130.0755, 81.9627) -> (130.6932, 81.4819) centre (148.5021, 105) ccw projected
  arc A423 (130.6932, 81.4819) -> (131.6176, 82.0318) centre (125.4951, 91.2714) ccw projected
  arc A424 (131.6176, 82.0318) -> (132.2472, 82.4915) centre (126.8777, 89.1849) ccw projected
  arc A425 (132.2472, 82.4915) -> (132.6446, 82.8391) centre (128.3619, 87.3348) ccw projected
  arc A426 (132.6446, 82.8391) -> (133.3084, 82.3788) centre (148.5021, 105) ccw projected
  arc A427 (133.3084, 82.3788) -> (133.1222, 81.8848) centre (139.0204, 79.9444) ccw projected
  arc A428 (133.1222, 81.8848) -> (132.9125, 81.1339) centre (141.2734, 79.2031) ccw projected
  arc A429 (132.9125, 81.1339) -> (132.7216, 80.0755) centre (143.7122, 78.6399) ccw projected
  arc A430 (132.7216, 80.0755) -> (133.3885, 79.6656) centre (148.5021, 105) ccw projected
  arc A431 (133.3885, 79.6656) -> (134.2467, 80.3138) centre (127.145, 88.8238) ccw projected
  arc A432 (134.2467, 80.3138) -> (134.822, 80.84) centre (128.7487, 86.902) ccw projected
  arc A433 (134.822, 80.84) -> (135.1787, 81.2291) centre (130.4274, 85.2264) ccw projected
  arc A434 (135.1787, 81.2291) -> (135.8891, 80.8447) centre (148.5021, 105) ccw projected
  arc A435 (135.8891, 80.8447) -> (135.7584, 80.3332) centre (141.8342, 79.0534) ccw projected
  arc A436 (135.7584, 80.3332) -> (135.6326, 79.5638) centre (144.1552, 78.5645) ccw projected
  arc A437 (135.6326, 79.5638) -> (135.5593, 78.4908) centre (146.6411, 78.273) ccw projected
  arc A438 (135.5593, 78.4908) -> (136.2672, 78.1567) centre (148.5021, 105) ccw projected
  arc A439 (136.2672, 78.1567) -> (137.0489, 78.8954) centre (129.0541, 86.5725) ccw projected
  arc A440 (137.0489, 78.8954) -> (137.5628, 79.4817) centre (130.8595, 84.8389) ccw projected
  arc A441 (137.5628, 79.4817) -> (137.8746, 79.9077) centre (132.7124, 83.3581) ccw projected
  arc A442 (137.8746, 79.9077) -> (138.623, 79.6038) centre (148.5021, 105) ccw projected
  arc A443 (138.623, 79.6038) -> (138.5493, 79.081) centre (144.729, 78.4773) ccw projected
  arc A444 (138.5493, 79.081) -> (138.5089, 78.3024) centre (147.0897, 78.2467) ccw projected
  arc A445 (138.5089, 78.3024) -> (138.5541, 77.2279) centre (149.5926, 78.2305) ccw projected
  arc A446 (138.5541, 77.2279) -> (139.2945, 76.9737) centre (148.5021, 105) ccw projected
  arc A447 (139.2945, 76.9737) -> (139.9902, 77.7939) centre (131.1993, 84.5449) ccw projected
  arc A448 (139.9902, 77.7939) -> (140.4364, 78.4331) centre (133.1845, 83.0204) ccw projected
  arc A449 (140.4364, 78.4331) -> (140.6994, 78.8909) centre (135.189, 81.7524) ccw projected
  arc A450 (140.6994, 78.8909) -> (141.4767, 78.6711) centre (148.5021, 105) ccw projected
  arc A451 (141.4767, 78.6711) -> (141.4611, 78.1434) centre (147.6697, 78.2232) ccw projected
  arc A452 (141.4611, 78.1434) -> (141.5065, 77.3651) centre (150.0413, 78.2537) ccw projected
  arc A453 (141.5065, 77.3651) -> (141.6696, 76.3021) centre (152.5309, 78.5129) ccw projected
  arc A454 (141.6696, 76.3021) -> (142.4335, 76.1309) centre (148.5021, 105) ccw projected
  arc A455 (142.4335, 76.1309) -> (143.0347, 77.0227) centre (133.5546, 82.7656) ccw projected
  arc A456 (143.0347, 77.0227) -> (143.4079, 77.7071) centre (135.6954, 81.4687) ccw projected
  arc A457 (143.4079, 77.7071) -> (143.619, 78.191) centre (137.8272, 80.429) ccw projected
  arc A458 (143.619, 78.191) -> (144.4157, 78.0581) centre (148.5021, 105) ccw projected
  arc A459 (144.4157, 78.0581) -> (144.4582, 77.5318) centre (150.6204, 78.2942) ccw projected
  arc A460 (144.4582, 77.5318) -> (144.589, 76.7633) centre (152.9743, 78.5854) ccw projected
  arc A461 (144.589, 76.7633) -> (144.8681, 75.7246) centre (155.4202, 79.1169) ccw projected
  arc A462 (144.8681, 75.7246) -> (145.6462, 75.6385) centre (148.5021, 105) ccw projected
  arc A463 (145.6462, 75.6385) -> (146.1456, 76.591) centre (136.0913, 81.2562) ccw projected
  arc A464 (146.1456, 76.591) -> (146.4413, 77.3123) centre (138.3618, 80.2027) ccw projected
  arc A465 (146.4413, 77.3123) -> (146.5978, 77.8165) centre (140.595, 79.4038) ccw projected
  arc A466 (146.5978, 77.8165) -> (147.4044, 77.772) centre (148.5021, 105) ccw projected
  arc A467 (147.4044, 77.772) -> (147.5045, 77.2537) centre (153.5454, 78.6893) ccw projected
  arc A468 (147.5045, 77.2537) -> (147.719, 76.5042) centre (155.853, 79.2377) ccw projected
  arc A469 (147.719, 76.5042) -> (148.1107, 75.5025) centre (158.2256, 80.035) ccw projected
  arc A470 (148.1107, 75.5025) -> (148.8935, 75.5025) centre (148.5021, 105) ccw projected
  circle A471 centre (148.5021, 105) radius 2.025 projected
  circle A472 centre (148.5021, 105) radius 5
  point P0 (0, 0)
  point P1 (151.9662, 107)
  point P2 (151.9662, 103)
  point P3 (148.5021, 101)
  point P4 (145.038, 103)
  point P5 (147.4196, 101.625)
  point P6 (150.8837, 102.375)
  point P7 (151.9662, 104.25)
  point P8 (151.9662, 105.75)
  point P9 (146.1205, 107.625)
  point P10 (145.038, 105.75)
  point P11 (146.1205, 102.375)
  dimension "d8" = 8
  dimension "d7" = 10
  dimension "d9" = 360
  dimension "d10" = 360
  dimension "d11" = 6.5263
  dimension "d12" = 1.5
  dimension "d13" = 1.25
  dimension "d18" = 10
  constraints: 30 point on circle, 15 centre point, 12 end point, 5 coincident, 2 point on line, 2 tangent, 1 vertical, 1 vertical alignment, 72 other
  measures "d7" diameter of A8
  measures "d11" diameter of A14
  measures "d12" radius of A11
  measures "d13" radius of A9
  measures "d18" diameter of A472
extrude "押し出し4" cut sketch "スケッチ2" against normal blind 3 contours A1 A2 A4 A3 A5 A12 A10 A6 A7 A9 A11 A0 | A8
extrude "押し出し5" add sketch "スケッチ2" against normal blind 2 contours A8
